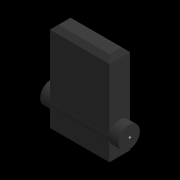
# Autodesk Inventor part: 40A_ATC_main_fuse
Saved by Autodesk Inventor 2020.2 (Build 242310000, 310)
## iProperties
Created: 2020-04-17
Part Number: 40A_ATC_main_fuse
Material: Rubber, Silicone
Document SubType Name: Modeling
Designer: agmlego
Mass: 15.5509 g
Surface Area: 39.5923 cm^2
Volume: 12.4407 cm^3
Density: 1.25 g/cm^3
Appearance: Rubber - Black
GlobalPropertyList: <PropertyList/>
Author: agmlego
Autodesk Inventor part; units mm, degrees
ref_plane "YZ Plane" through (0, 0, 0) normal (1, 0, 0) x (0, 1, 0)
ref_plane "XZ Plane" through (0, 0, 0) normal (0, 1, 0) x (-1, 0, 0)
ref_plane "XY Plane" through (0, 0, 0) normal (0, 0, 1) x (1, 0, 0)
sketch "Sketch1" plane through (0, 0, 0) normal (0, 0, 1) x (1, 0, 0)
  line L0 (0, 0) -> (28, 0)
  line L1 (28, 0) -> (28, 44)
  line L2 (28, 44) -> (0, 44)
  line L3 (0, 44) -> (0, 0)
  dimension "d0" = 44
  dimension "d1" = 28
  constraints: 8 end point, 2 parallel, 1 horizontal, 1 perpendicular
  measures "d0" distance of L2.end L0.start
  measures "d1" distance of L0.start L0.end
extrude "Extrusion1" add sketch "Sketch1" along normal blind 9.75
sketch "Sketch2" plane through (28, 0, 0) normal (1, 0, 0) x (0, 0, -1)
  circle A0 centre (-4.875, 12) radius 5
  line L0 (0, 0) -> (-9.75, 0) construction
  line L1 (-4.875, 0) -> (-4.875, 12) construction
  dimension "d4" = 10
  dimension "d5" = 12
  constraints: 2 end point, 1 centre point, 1 midpoint, 1 perpendicular
  measures "d4" diameter of A0
  measures "d5" distance of L1.start L1.end
extrude "Extrusion2" add sketch "Sketch2" along normal blind 4.45 and the other way blind 32.45
chamfer "Chamfer1" distance 2 angle 45 8 edges at (14, 44, 9.75) (14, 44, 0) (28, 44, 4.875) (0, 44, 4.875) (14, 0, 9.75) (0, 0, 4.875) (14, 0, 0) (28, 0, 4.875)
sketch "Sketch3" plane through (32.45, 12, 4.875) normal (1, 0, 0) x (0, 0, -1)
  circle A0 centre (0, 0) radius 5 construction
sketch "Sketch4" plane through (-4.45, 12, 4.875) normal (-1, 0, 0) x (0, 0, 1)
  circle A0 centre (0, 0) radius 5 construction
body "Solid1"
